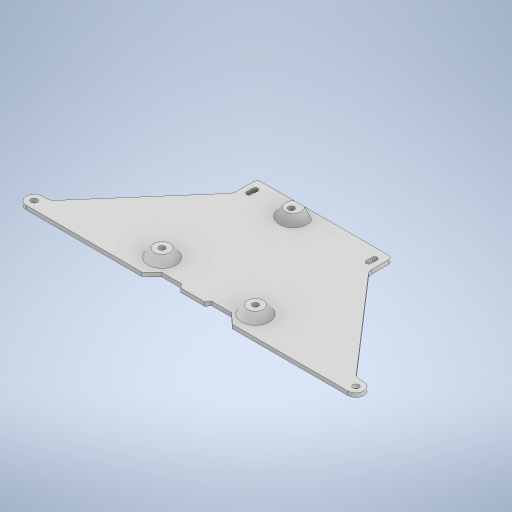
# Autodesk Inventor part: ArduSimple BasePlate FrontExit
Saved by Autodesk Inventor 2023 (Build 270158000, 158)
## iProperties
Created: 2022-12-11
Part Number: ArduSimple BasePlate FrontExit
Material: Generic
Document SubType Name: Modeling
Designer: Administrator
Density: 1 g/cm^3
Appearance: Default
Author: Administrator
Autodesk Inventor part; units mm, degrees
ref_plane "YZ Plane" through (0, 0, 0) normal (1, 0, 0) x (0, 1, 0)
ref_plane "XZ Plane" through (0, 0, 0) normal (0, 1, 0) x (-1, 0, 0)
ref_plane "XY Plane" through (0, 0, 0) normal (0, 0, 1) x (1, 0, 0)
sketch "Sketch1" plane through (0, 0, 0) normal (0, 1, 0) x (-1, 0, 0)
  circle A0 centre (-13, 3.6355) radius 1.25
  circle A1 centre (47, 3.6355) radius 1.25
  circle A2 centre (-63.9, 60.95) radius 1.55
  circle A3 centre (-63.9, 60.95) radius 1.5
  circle A4 centre (97.9, 60.95) radius 1.55
  circle A5 centre (97.9, 60.95) radius 1.5
  arc A6 (47, -0.3645) -> (51, 3.6355) centre (47, 3.6355) ccw construction
  arc A7 (-17, 3.6395) -> (-13, -0.3645) centre (-13, 3.6355) ccw construction
  arc A8 (-63.9, 64.95) -> (-63.9, 56.95) centre (-63.9, 60.95) ccw
  arc A9 (97.9, 56.95) -> (97.9, 64.95) centre (97.9, 60.95) ccw
  line L0 (-13, -0.3645) -> (47, -0.3645) construction
  line L1 (-63.9, 64.95) -> (97.9, 64.95)
  line L2 (-17, 3.6395) -> (-17, 6.1391)
  line L3 (51, 3.6355) -> (51, 6.1391)
  arc A10 (51, 3.6355) -> (47, -0.3645) centre (47, 3.6355) ccw construction
  arc A11 (-13, -0.3645) -> (-17, 3.6395) centre (-13, 3.6355) ccw construction
  line L4 (-63.9, 56.95) -> (-61.722, 56.95)
  line L5 (97.9, 56.95) -> (95.722, 56.95)
  line L6 (92.7041, 55.5753) -> (51.9821, 8.7645)
  line L7 (-58.7041, 55.5753) -> (-17.9821, 8.7645)
  arc A12 (-58.7041, 55.5753) -> (-61.722, 56.95) centre (-61.722, 52.95) ccw
  arc A13 (95.722, 56.95) -> (92.7041, 55.5753) centre (95.722, 52.95) ccw
  arc A14 (51.9821, 8.7645) -> (51, 6.1391) centre (55, 6.1391) ccw
  arc A15 (-17, 6.1391) -> (-17.9821, 8.7645) centre (-21, 6.1391) ccw
  arc A16 (-63.9, 56.95) -> (-63.9, 64.95) centre (-63.9, 60.95) ccw construction
  arc A17 (97.9, 64.95) -> (97.9, 56.95) centre (97.9, 60.95) ccw construction
  line L8 (51, 3.6355) -> (51, -2.3645)
  line L9 (49, -4.3645) -> (-15, -4.3645)
  line L10 (-17, -2.3645) -> (-17, 3.6395)
  arc A18 (49, -4.3645) -> (51, -2.3645) centre (49, -2.3645) ccw
  arc A19 (-17, -2.3645) -> (-15, -4.3645) centre (-15, -2.3645) ccw
  line L11 (-13, 3.6355) -> (-13, 0.6355) construction
  line L12 (-14.25, 3.6355) -> (-14.25, 0.6355)
  line L13 (-11.75, 0.6355) -> (-11.75, 3.6355)
  arc A20 (-11.75, 3.6355) -> (-14.25, 3.6355) centre (-13, 3.6355) ccw
  arc A21 (-14.25, 0.6355) -> (-11.75, 0.6355) centre (-13, 0.6355) ccw
  line L14 (47, 3.6355) -> (47, 0.6355) construction
  line L15 (45.75, 3.6355) -> (45.75, 0.6355)
  line L16 (48.25, 0.6355) -> (48.25, 3.6355)
  arc A22 (48.25, 3.6355) -> (45.75, 3.6355) centre (47, 3.6355) ccw
  arc A23 (45.75, 0.6355) -> (48.25, 0.6355) centre (47, 0.6355) ccw
  point P0 (0, 0)
  point P1 (17, 90.5)
  point P2 (51, -4.3645)
  point P3 (-13, 2.1355)
  point P4 (47, 2.1355)
  point P5 (-11.75, 3.6355)
  dimension "d0" = 2.5
  dimension "d1" = 2.5
  dimension "d2" = 3
  dimension "d3" = 3
  dimension "d4" = 8
  dimension "d5" = 8
  dimension "d6" = 8
  dimension "d7" = 8
  dimension "d8" = 60
  dimension "d18" = 4
  dimension "d313" = 8
  dimension "d314" = 2
  dimension "d322" = 3
  dimension "d323" = 3
  constraints: 38 end point, 36 point on circle, 24 centre point, 24 tangent, 5 coincident, 5 equal radius, 4 vertical, 3 parallel, 2 horizontal, 2 midpoint, 2 perpendicular, 2 point on line
  measures "d0" diameter of A0
  measures "d1" diameter of A1
  measures "d2" diameter of A3
  measures "d3" diameter of A5
  measures "d4" diameter of A6
  measures "d5" diameter of A7
  measures "d6" diameter of A8
  measures "d7" diameter of A9
  measures "d8" distance of A1.centre A0.centre
  measures "d18" radius of A12
  measures "d313" distance of L3.start point (51, -4.365)
  measures "d314" radius of A18
  measures "d322" distance of L11.start L11.end
  measures "d323" distance of L14.start L14.end
extrude "Extrusion1" add sketch "Sketch1" along normal blind 2 contours L1 A9 L5 A13 L6 A14 L3 L8 A18 L9 A19 L10 L2 A15 L7 A12 L4 A8
sketch "Sketch3" plane through (0, 2, 0) normal (0, 1, 0) x (1, 0, 0)
  circle A0 centre (13, -3.6355) radius 1.55 construction
  line L0 (13, -3.6355) -> (-2, 2) construction
  line L1 (-2, 2) -> (-2, 4) construction
  line L2 (-2, 2) -> (-2, 4) construction
  line L3 (-2, 4) -> (6, 6.8723) construction
  line L4 (9.8, 6.8723) -> (53.9673, -18.6277) construction
  line L5 (6, 6.8723) -> (9.8, 6.8723) construction
  line L6 (9.8, 6.8723) -> (53.9673, -18.6277) construction
  line L7 (57.4673, -24.6899) -> (57.0036, -33.6779) construction
  line L8 (53.9673, -18.6277) -> (57.4673, -24.6899) construction
  line L9 (57.4673, -24.6899) -> (57.0036, -33.6779) construction
  line L10 (75.376, -65.5) -> (80.5, -65.5) construction
  line L11 (57.0036, -33.6779) -> (75.376, -65.5) construction
  line L12 (75.376, -65.5) -> (6.5, -65.7) construction
  line L13 (6.5, -65.7) -> (6.2893, -65.5) construction
  line L14 (0.6, -60.1) -> (-9.5, -60.1)
  line L15 (-9.5, -60.1) -> (-11, -62.1)
  line L16 (-9.5, -60.1) -> (-11, -62.1)
  line L17 (-23, -62.1) -> (-11, -62.1)
  line L18 (-11, -62.1) -> (-23, -62.1)
  line L19 (-24.5, -60.1) -> (-23, -62.1)
  line L20 (-23, -62.1) -> (-24.5, -60.1)
  line L21 (-34.6, -60.1) -> (-24.5, -60.1)
  line L22 (-24.5, -60.1) -> (-34.6, -60.1)
  line L23 (-40.5, -71.9) -> (-40.5, -65.7) construction
  line L24 (-34.6, -60.1) -> (-39.7098, -64.95)
  line L25 (-114.5, -65.5) -> (-109.376, -65.5) construction
  line L26 (-40.5, -65.7) -> (-109.376, -65.5) construction
  line L27 (-109.376, -65.5) -> (-91.0036, -33.6779) construction
  line L28 (-87.9673, -18.6277) -> (-91.4673, -24.6899) construction
  line L29 (-91.0036, -33.6779) -> (-91.4673, -24.6899) construction
  line L30 (-91.4673, -24.6899) -> (-87.9673, -18.6277) construction
  line L31 (-40, 6.8723) -> (-43.8, 6.8723) construction
  line L32 (-87.9673, -18.6277) -> (-43.8, 6.8723) construction
  line L33 (-43.8, 6.8723) -> (-40, 6.8723) construction
  line L34 (-32, 4) -> (-40, 6.8723) construction
  line L35 (-40, 6.8723) -> (-32, 4) construction
  line L36 (-32, 4) -> (-32, 2) construction
  line L37 (-32, 2) -> (-2, 2) construction
  line L38 (-6.4, -15.5) -> (-2.8831, -15.5)
  line L39 (-2.8831, -15.5) -> (-6.4, -15.5)
  line L40 (-26.1, -17.5) -> (-7.9, -17.5)
  line L41 (-6.4, -15.5) -> (-7.9, -17.5)
  line L42 (-7.9, -17.5) -> (-26.1, -17.5)
  line L43 (-31.1169, -15.5) -> (-27.6, -15.5)
  line L44 (-26.1, -17.5) -> (-27.6, -15.5)
  line L45 (-35.1306, -20.7029) -> (-31.1169, -15.5)
  line L46 (-27.6, -15.5) -> (-31.1169, -15.5)
  line L47 (-31.1169, -15.5) -> (-35.1306, -20.7029)
  line L48 (-35.1306, -20.7029) -> (-27.0449, -36)
  line L49 (-22.7189, -36) -> (-27.0449, -36)
  line L50 (-27.0449, -36) -> (-22.7189, -36)
  line L51 (-20.9689, -37) -> (-22.7189, -36)
  line L52 (-22.7189, -36) -> (-20.9689, -37)
  line L53 (-13.0311, -37) -> (-20.9689, -37)
  line L54 (-20.9689, -37) -> (-13.0311, -37)
  line L55 (-11.2811, -36) -> (-13.0311, -37)
  line L56 (-13.0311, -37) -> (-11.2811, -36)
  line L57 (-6.9551, -36) -> (-11.2811, -36)
  line L58 (-11.2811, -36) -> (-6.9551, -36)
  line L59 (1.1306, -20.7029) -> (-6.9551, -36)
  line L60 (-6.9551, -36) -> (1.1306, -20.7029)
  line L61 (1.1306, -20.7029) -> (-2.8831, -15.5)
  arc A1 (11.75, -3.6355) -> (14.25, -3.6355) centre (13, -3.6355) ccw projected
  line L62 (-97.9, -64.95) -> (63.9, -64.95) projected
  line L63 (5.7098, -64.95) -> (-39.7098, -64.95)
  line L64 (5.7098, -64.95) -> (0.6, -60.1)
  point P0 (0, 0)
  point P1 (17, 90.5)
  constraints: 128 end point, 15 collinear, 5 perpendicular, 4 parallel, 3 point on line, 1 centre point, 1 coincident
extrude "Extrusion3" cut sketch "Sketch3" against normal up to next contours L64 L62 L24 L21 L19 L17 L15 L14
sketch "Sketch16" plane through (0, 0, 0) normal (0, -1, 0) x (1, 0, 0)
  line L0 (-34.6, 60.1) -> (-39.7098, 64.95) construction
  line L1 (-34.6, 60.1) -> (-34.6, 54) construction
  line L2 (-34.6, 54) -> (-38.1, 54) construction
  circle A0 centre (-38.1, 54) radius 3
  circle A1 centre (4.1, 54) radius 3
  line L3 (0.6, 60.1) -> (-9.5, 60.1) construction
  point P0 (0, 0)
  dimension "d114" = 6.1
  dimension "d115" = 3.5
  dimension "d116" = 6
  dimension "d117" = 6
  dimension "d118" = 42.2
  dimension "d119" = 6.1
  constraints: 4 end point, 2 centre point, 1 coincident, 1 perpendicular, 1 vertical
  measures "d114" distance of L0.start L1.end
  measures "d115" distance of L1.end L2.end
  measures "d116" diameter of A0
  measures "d117" diameter of A1
  measures "d118" distance of A1.centre L2.end
  measures "d119" distance from line of A1.centre L3
sketch "Sketch2" plane through (0, 2, 0) normal (0, 1, 0) x (1, 0, 0)
  arc A0 (11.75, -3.6355) -> (14.25, -3.6355) centre (13, -3.6355) ccw projected
  arc A1 (-48.25, -3.6355) -> (-45.75, -3.6355) centre (-47, -3.6355) ccw projected
  line L0 (13, 0.3645) -> (-47, 0.3645) projected
  circle A2 centre (-41.13, -53.4355) radius 4
  circle A3 centre (7.13, -54.7055) radius 4
  circle A4 centre (-25.89, -2.6355) radius 4
  point P0 (0, 0)
  point P1 (-28.5358, 0.3645)
  point P2 (-23.2442, 0.3645)
  dimension "d21" = 60
  dimension "d337" = 8
  dimension "d343" = 8
  dimension "d345" = 48.26
  dimension "d346" = 5.87
  dimension "d348" = 1.27
  dimension "d349" = 8
  dimension "d350" = 1
  dimension "d351" = 15.24
  dimension "d352" = 50.8
  constraints: 3 centre point
  measures "d21" distance of A0.centre A1.centre
  measures "d337" diameter of A2
  measures "d343" diameter of A3
  measures "d345" horizontal distance of A3.centre A2.centre
  measures "d346" horizontal distance of A0.centre A3.centre
  measures "d348" vertical distance of A3.centre A2.centre
  measures "d349" diameter of A4
  measures "d350" vertical distance of A0.centre A4.centre
  measures "d351" horizontal distance of A2.centre A4.centre
  measures "d352" vertical distance of A4.centre A2.centre
extrude "Extrusion2" add sketch "Sketch2" along normal blind 4 contours A4 L0 | A2 | A3 picked at (-26.9026, -3.4826)
chamfer "Chamfer2" distance 3 distance2 4 3 edges at (-45.13, 2, 53.4355) (3.13, 2, 54.7055) (-25.89, 2, 6.6355) measured on face at (2.63, 2, 54.7055) measured on face at (-25.89, 2, 7.1355) measured on face at (-45.63, 2, 53.4355)
sketch "Sketch17" plane through (0, 2, 0) normal (0, 1, 0) x (1, 0, 0)
  arc A0 (11.75, -3.6355) -> (14.25, -3.6355) centre (13, -3.6355) ccw projected
  circle A1 centre (13, -3.6355) radius 2.5
  arc A2 (-48.25, -3.6355) -> (-45.75, -3.6355) centre (-47, -3.6355) ccw projected
  circle A3 centre (-47, -3.6355) radius 2.5
  line L0 (13, -3.6355) -> (13, 0) construction
  line L1 (15.5, -3.6355) -> (15.5, 0)
  line L2 (10.5, 0) -> (10.5, -3.6355)
  arc A4 (10.5, -3.6355) -> (15.5, -3.6355) centre (13, -3.6355) ccw
  arc A5 (15.5, 0) -> (10.5, 0) centre (13, 0) ccw
  line L3 (-47, -3.6355) -> (-47, 0) construction
  line L4 (-44.5038, -3.6355) -> (-44.5038, 0)
  line L5 (-49.4962, 0) -> (-49.4962, -3.6355)
  arc A6 (-49.4962, -3.6355) -> (-44.5038, -3.6355) centre (-47, -3.6355) ccw
  arc A7 (-44.5038, 0) -> (-49.4962, 0) centre (-47, 0) ccw
  point P0 (0, 0)
  point P1 (13, -1.8177)
  point P2 (-47, -1.8177)
  point P3 (-49.4962, -3.4982)
  point P4 (-44.5038, -3.4982)
  dimension "d125" = 5
  dimension "d126" = 5
  constraints: 16 end point, 8 point on circle, 8 tangent, 6 centre point, 3 parallel, 2 coincident, 2 midpoint, 1 concentric, 1 vertical
  measures "d125" diameter of A1
  measures "d126" diameter of A3
extrude "Extrusion17" cut sketch "Sketch17" along normal through all
extrude "Extrusion18" cut sketch "Sketch16" against normal blind 2
sketch "Sketch22" plane through (-39.5, 6, 6.6355) normal (0, 1, 0) x (1, 0, 0)
  circle A0 centre (13.61, 3) radius 1.5
  circle A1 centre (13.61, 3) radius 4 projected
  circle A2 centre (-1.63, -46.8) radius 4 projected
  circle A3 centre (-1.63, -46.8) radius 1.5
  circle A4 centre (46.63, -48.07) radius 4 projected
  circle A5 centre (46.63, -48.07) radius 1.5
  dimension "d168" = 3
  dimension "d339" = 3
  dimension "d347" = 3
  constraints: 3 centre point, 2 coincident, 1 concentric
  measures "d168" diameter of A0
  measures "d339" diameter of A3
  measures "d347" diameter of A5
extrude "Extrusion24" cut sketch "Sketch22" against normal blind 5 contours A0 | A3 | A5
body "Solid1"
